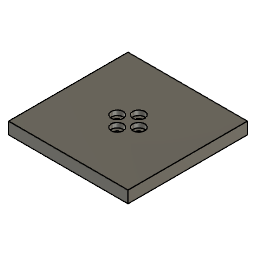
Simple Motor Mount (Autodesk Fusion 360 design; units mm, degrees)
Autodesk Fusion 360 part; units mm, degrees
sketch "Sketch1" plane through (0, 0, 0) normal (0, 0, 1) x (1, 0, 0)
  line L0 (-25, 25) -> (25, 25)
  line L1 (25, 25) -> (25, -25)
  line L2 (25, -25) -> (-25, -25)
  line L3 (-25, -25) -> (-25, 25)
  constraint horizontal L0
  constraint vertical L1
  constraint horizontal L2
  constraint vertical L3
extrude "Extrude1" add sketch "Sketch1" along normal blind 5
sketch "Sketch2" plane through (0, 0, 5) normal (0, 0, 1) x (-1, 0, 0)
  line L0 (25, 25) -> (-25, 25)
  line L1 (-25, 25) -> (-25, -25)
  line L2 (-25, -25) -> (25, -25)
  line L3 (25, -25) -> (25, 25)
  circle A0 centre (0, 0) radius 4.5
  line L4 (0.0733, -4.4994) -> (0.0733, 4.4994)
  line L5 (4.5, 0) -> (-4.5, 0)
  dimension "d3" = 9
  constraint coincident A0.centre origin
  constraint coincident A0 L4.start
  constraint coincident A0 L4.end
  constraint parallel L3 L4
  constraint coincident A0 L5.start
  constraint coincident A0 L5.end
  constraint perpendicular L4 L5
  measures "d3" diameter of A0
hole "Hole1" at (-4.5, 0, 5) direction (0, 0, -1) diameter 2.1 depth 11 tip angle 118 counterbore diameter 5 counterbore depth 2
pattern_circular "C-Pattern1" count 4 over 360 about axis through (0, 0, 1.75) along (0, 0, 1) of "Hole1"
extrude "Extrude2" add 1 faces at (-18.5157, 0.0262, 0) along direction (0, 0, -1) blind 2
extrude "Extrude3" cut 1 faces at (-18.5157, 0.0262, -2) along direction (0, 0, 1) blind 2
